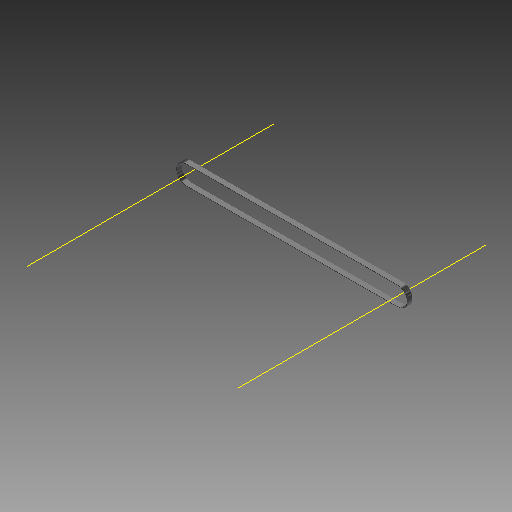
# Autodesk Inventor part: Synchronous Belt
Saved by Autodesk Inventor 2017 (Build 210142000, 142)
## iProperties
Created: 2017-11-17
Part Number: Synchronous Belt
Material: Rubber
Document SubType Name: Modeling
Designer: Biscuit
Density: 1 g/cm^3
Appearance: Rubber - Black - Version 1.1
CustomPartVersion: 1
Author: Biscuit
Autodesk Inventor part; units mm, degrees
ref_plane "YZ Plane" through (0, 0, 0) normal (1, 0, 0) x (0, 1, 0)
ref_plane "XZ Plane" through (0, 0, 0) normal (0, 1, 0) x (-1, 0, 0)
ref_plane "XY Plane" through (0, 0, 0) normal (0, 0, 1) x (1, 0, 0)
sketch "Sketch Path" plane through (0, 0, 0) normal (0, 0, 1) x (1, 0, 0)
  arc A0 (19.9523, -20.2064) -> (20.0477, -42.4879) centre (20, -31.3472) ccw
  arc A1 (270.5477, -41.4156) -> (270.4523, -19.1341) centre (270.5, -30.2749) ccw
  line L0 (270.5477, -41.4156) -> (20.0477, -42.4879)
  line L1 (19.9523, -20.2064) -> (270.4523, -19.1341)
  point P0 (10.0164, 35.326)
  point P1 (9.9836, 27.3683)
  point P2 (270.4836, 26.296)
  point P3 (270.5164, 34.2537)
  point P4 (9.9836, -27.3683)
  point P5 (10.0164, -35.326)
  point P6 (270.5164, -34.2537)
  point P7 (270.4836, -26.296)
  point P8 (20.2708, -20.2096)
  point P9 (20.3662, -42.482)
  point P10 (270.6308, -34.2516)
  point P11 (270.5967, -26.2972)
  constraints: 4 end point, 4 point on circle, 2 centre point
ref_plane "Cross Section Plane" through (20.0477, -42.4879, 0) normal (0.9999908, 0.0042805, 0) x (0, 0, 1)
ref_plane "Work Plane2" through (20, -31.3472, 0) normal (-1, 0, 0) x (0, 0, 1)
ref_plane "Work Plane3" through (270.5, -30.2749, 0) normal (-0.9839664, 0.1783542, 0) x (0, 0, 1)
ref_plane "Work Plane4" through (20, -42.488, 0) normal (0, 0, -1) x (-1, 0, 0)
sketch3d "Sketch3"
  constraints: 13 end point, 3 parallel, 2 midpoint, 2 perpendicular, 2 point on line, 1 horizontal alignment, 1 vertical, 1 other
feature "iSBeltToothT:1" [suppressed]
pattern_linear "Rectangular Pattern1" [suppressed]
sketch "Cross Section" plane through (20.0477, -42.4879, 0) normal (0.9999908, 0.0042805, 0) x (0, 0, 1)
  line L0 (-3, 0.3) -> (3, 0.3)
  line L1 (3, 0.3) -> (3, -0.3)
  line L2 (3, -0.3) -> (-3, -0.3)
  line L3 (-3, -0.3) -> (-3, 0.3)
  line L4 (-3, 0) -> (3, 0) construction
  point P0 (0, 0)
  point P1 (0, 0)
  dimension "d0" = 6
  dimension "d4" = 0.3
  dimension "d5" = 0.3
  constraints: 10 end point, 3 midpoint, 2 parallel, 1 coincident, 1 horizontal, 1 perpendicular, 1 other
  measures "d0" distance between parallel lines of L1 L3
  measures "d4" distance between parallel lines of L2 L4
  measures "d5" distance between parallel lines of L4 L0
sweep "Belt" add profiles "Cross Section" path "Sketch Path" path curves L1 A1 L0 A0
fillet "Fillet1" [suppressed]
equation "\"d0\" = da_B"
equation "\"d4\" = da_a"
equation "\"d5\" = da_a2"
equation "\"d21\" = d13"
equation "\"d20\" = da_pb"
equation "\"da_B\" = 6"
equation "\"da_pb\" = 2.5"
equation "\"da_L\" = 571.00459"
equation "\"da_a\" = 0.3"
equation "\"da_S\" = 1.5"
equation "\"da_Beta\" = 20deg"
equation "\"da_Ht\" = 0.7"
equation "\"da_H\" = 1.3"
equation "\"da_a2\" = 0.3"
equation "\"d13\" = 0.2"
body "Solid1"
